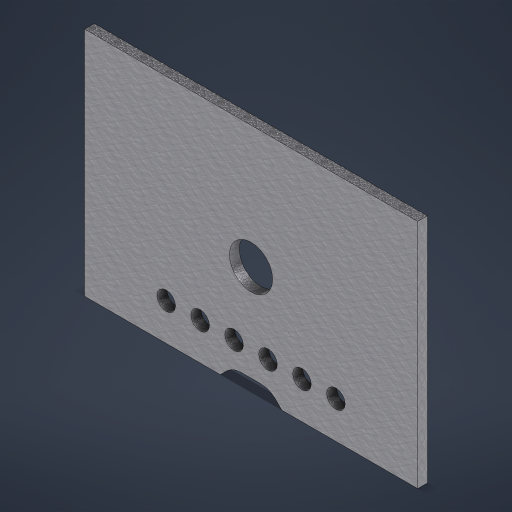
# Autodesk Inventor part: ArmSupportPlate
Saved by Autodesk Inventor 2024 (Build 280153000, 153)
## iProperties
Created: 2023-11-22
Part Number: ArmSupportPlate
Material: Generic
Document SubType Name: Modeling
Designer: avsar
Density: 1 g/cm^3
Appearance: Machined 02
Author: avsar
Autodesk Inventor part; units mm, degrees
ref_plane "YZ Plane" through (0, 0, 0) normal (1, 0, 0) x (0, 1, 0)
ref_plane "XZ Plane" through (0, 0, 0) normal (0, 1, 0) x (-1, 0, 0)
ref_plane "XY Plane" through (0, 0, 0) normal (0, 0, 1) x (1, 0, 0)
sketch "Sketch1" plane through (0, 0, 0) normal (0, 0, 1) x (1, 0, 0)
  line L0 (-54, -37.5) -> (54, -37.5)
  line L1 (54, -37.5) -> (54, 37.5)
  line L2 (54, 37.5) -> (-54, 37.5)
  line L3 (-54, 37.5) -> (-54, -37.5)
  line L4 (-54, -37.5) -> (54, 37.5) construction
  line L5 (54, -37.5) -> (-54, 37.5) construction
  point P0 (0, 0)
  dimension "d0" = 108
  dimension "d1" = 75
  constraints: 12 end point, 2 midpoint, 2 parallel, 1 horizontal, 1 perpendicular
  measures "d0" distance of L2.end L1.end
  measures "d1" distance of L1.end L0.end
extrude "Extrusion1" add sketch "Sketch1" along normal mid plane 3.175
sketch "Sketch3" plane through (0, 0, 1.5875) normal (0, 0, 1) x (1, 0, 0)
  line L0 (-54, -37.5) -> (54, -37.5) construction
  line L1 (-10, -37.5) -> (-6, -33.5)
  line L2 (-6, -33.5) -> (6, -33.5)
  line L3 (6, -33.5) -> (10, -37.5)
  line L4 (-10, -37.5) -> (10, -37.5)
  point P0 (0, 0)
  point P1 (0, -33.5)
  point P2 (0, -37.5)
  dimension "d16" = 12
  dimension "d17" = 4
  dimension "d18" = 45
  constraints: 8 end point, 2 midpoint, 2 point on line, 1 collinear, 1 parallel, 1 perpendicular, 1 vertical alignment
  measures "d16" distance of L1.end L2.end
  measures "d17" distance from line of point (0, -37.5) L2
  measures "d18" angle of L0 L3
extrude "Extrusion3" cut sketch "Sketch3" against normal through all
fillet "Fillet1" radius 6.5 2 edges at (-6, -33.5, 0) (6, -33.5, 0)
sketch "Sketch4" plane through (0, 0, 1.5875) normal (0, 0, 1) x (1, 0, 0)
  circle A0 centre (0, -2.325) radius 7
  line L0 (10, -37.5) -> (54, -37.5) construction
  point P0 (0, 0)
  dimension "d22" = 14
  dimension "d23" = 35.175
  constraints: 1 centre point, 1 vertical alignment
  measures "d22" diameter of A0
  measures "d23" distance from line of L0 A0.centre
extrude "Extrusion4" cut sketch "Sketch4" against normal through all
sketch "Sketch5" plane through (0, 0, 1.5875) normal (0, 0, 1) x (1, 0, 0)
  circle A0 centre (-27.5, -25.5) radius 3
  line L0 (-54, -37.5) -> (-10, -37.5) construction
  circle A1 centre (-16.5, -25.5) radius 3
  circle A2 centre (-5.5, -25.5) radius 3
  circle A3 centre (5.5, -25.5) radius 3
  circle A4 centre (16.5, -25.5) radius 3
  circle A5 centre (27.5, -25.5) radius 3
  line L1 (-5.5, -25.5) -> (5.5, -25.5) construction
  point P0 (0, 0)
  point P1 (0, -25.5)
  dimension "d26" = 6
  dimension "d27" = 12
  dimension "d30" = 11
  constraints: 6 centre point, 2 end point, 2 horizontal, 1 midpoint, 1 vertical alignment, 10 other
  measures "d26" diameter of A0
  measures "d27" distance from line of L0 A0.centre
  measures "d30" distance of A0.centre A1.centre
extrude "Extrusion5" cut sketch "Sketch5" against normal blind 10
body "Solid1"
